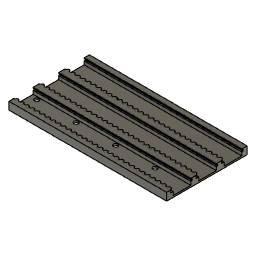
Plate Feeder for larger components v47 (Autodesk Fusion 360 design; units mm, degrees)
Autodesk Fusion 360 part; units mm, degrees
note: some values were not read from the file. Set by a fixed rule: which sketch regions a step uses.
sketch "Front view" plane through (0, 0, 0) normal (1, 0, 0) x (0, 1, 0)
  line L0 (0, 0) -> (16.4, 0)
  line L1 (16.4, 0) -> (16.4, 1.2)
  line L2 (16.4, 1.2) -> (0, 1.2)
  line L3 (0, 1.2) -> (0, 0)
  line L4 (0, 0) -> (-3, 0)
  line L5 (-3, 0) -> (-3, 5.8)
  line L6 (-3, 5.8) -> (0, 5.8)
  line L7 (0, 5.8) -> (0, 0)
  line L8 (16.4, 0) -> (19.4, 0)
  line L9 (19.4, 0) -> (19.4, 5.8)
  line L10 (19.4, 5.8) -> (16.4, 5.8)
  line L11 (16.4, 5.8) -> (16.4, 0)
  line L12 (0, 1.2) -> (16.4, 1.2)
  line L13 (16.4, 1.2) -> (16.4, 4.2) construction
  line L14 (16.4, 4.2) -> (0, 4.2) construction
  line L15 (0, 4.2) -> (0, 1.2) construction
  line L16 (16.4, 1.2) -> (15.4, 1.2)
  line L17 (15.4, 1.2) -> (15.4, 3.8)
  line L18 (15.4, 3.8) -> (16.4, 3.8)
  line L19 (16.4, 3.8) -> (16.4, 1.2)
  line L20 (0, 1.2) -> (2, 1.2)
  line L21 (2, 1.2) -> (2, 3.8)
  line L22 (2, 3.8) -> (0, 3.8)
  line L23 (0, 3.8) -> (0, 1.2)
  line L24 (35.8, 0) -> (35.8, 1.2)
  line L25 (35.8, 4.2) -> (19.4, 4.2) construction
  line L26 (35.8, 1.2) -> (34.8, 1.2)
  line L27 (35.8, 1.2) -> (35.8, 4.2) construction
  line L28 (34.8, 1.2) -> (34.8, 3.8)
  line L29 (21.4, 3.8) -> (19.4, 3.8)
  line L30 (38.8, 0) -> (38.8, 5.8)
  line L31 (19.4, 1.2) -> (21.4, 1.2)
  line L32 (21.4, 1.2) -> (21.4, 3.8)
  line L33 (35.8, 0) -> (38.8, 0)
  line L34 (34.8, 3.8) -> (35.8, 3.8)
  line L35 (35.8, 3.8) -> (35.8, 1.2)
  line L36 (38.8, 5.8) -> (35.8, 5.8)
  line L37 (35.8, 5.8) -> (35.8, 0)
  line L38 (35.8, 1.2) -> (19.4, 1.2)
  line L39 (19.4, 1.2) -> (35.8, 1.2)
  line L40 (19.4, 0) -> (35.8, 0)
  line L41 (55.2, 0) -> (55.2, 1.2)
  line L42 (55.2, 4.2) -> (38.8, 4.2) construction
  line L43 (55.2, 1.2) -> (54.2, 1.2)
  line L44 (55.2, 1.2) -> (55.2, 4.2) construction
  line L45 (54.2, 1.2) -> (54.2, 3.8)
  line L46 (40.8, 3.8) -> (38.8, 3.8)
  line L47 (58.2, 0) -> (58.2, 5.8)
  line L48 (38.8, 1.2) -> (40.8, 1.2)
  line L49 (40.8, 1.2) -> (40.8, 3.8)
  line L50 (55.2, 0) -> (58.2, 0)
  line L51 (54.2, 3.8) -> (55.2, 3.8)
  line L52 (55.2, 3.8) -> (55.2, 1.2)
  line L53 (58.2, 5.8) -> (55.2, 5.8)
  line L54 (55.2, 5.8) -> (55.2, 0)
  line L55 (55.2, 1.2) -> (38.8, 1.2)
  line L56 (38.8, 1.2) -> (55.2, 1.2)
  line L57 (38.8, 0) -> (55.2, 0)
  line L58 (0, 5.8) -> (2, 5.8)
  line L59 (2, 5.8) -> (2, 5.2)
  line L60 (2, 5.2) -> (0, 5.2)
  line L61 (0, 5.2) -> (0, 5.8)
  line L62 (16.4, 5.8) -> (15.4, 5.8)
  line L63 (15.4, 5.8) -> (15.4, 5.2)
  line L64 (15.4, 5.2) -> (16.4, 5.2)
  line L65 (16.4, 5.2) -> (16.4, 5.8)
  line L66 (34.8, 5.8) -> (34.8, 5.2)
  line L67 (35.8, 5.2) -> (35.8, 5.8)
  line L68 (35.8, 5.8) -> (34.8, 5.8)
  line L69 (34.8, 5.2) -> (35.8, 5.2)
  line L70 (21.4, 5.2) -> (19.4, 5.2)
  line L71 (19.4, 5.8) -> (21.4, 5.8)
  line L72 (21.4, 5.8) -> (21.4, 5.2)
  line L73 (54.2, 5.8) -> (54.2, 5.2)
  line L74 (55.2, 5.2) -> (55.2, 5.8)
  line L75 (55.2, 5.8) -> (54.2, 5.8)
  line L76 (54.2, 5.2) -> (55.2, 5.2)
  line L77 (40.8, 5.2) -> (38.8, 5.2)
  line L78 (38.8, 5.8) -> (40.8, 5.8)
  line L79 (40.8, 5.8) -> (40.8, 5.2)
  dimension "d8" = 16.4
  dimension "d9" = 1.2
  dimension "d11" = 3
  dimension "d12" = 5.8
  dimension "d14" = 3
  dimension "d15" = 5.8
  dimension "d17" = 16.4
  dimension "d18" = 3
  dimension "d20" = 1
  dimension "d21" = 2.6
  dimension "d22" = 2
  dimension "d23" = 2.6
  dimension "d33" = 38.8
  dimension "d34" = 0
  dimension "d65" = 2
  dimension "d66" = 0.6
  dimension "d67" = 1
  dimension "d68" = 0.6
  constraint horizontal L0
  constraint vertical L1
  constraint horizontal L2
  constraint vertical L3
  constraint coincident L0.start L3.end
  constraint horizontal L4
  constraint vertical L5
  constraint horizontal L6
  constraint vertical L7
  constraint horizontal L8
  constraint vertical L9
  constraint horizontal L10
  constraint vertical L11
  constraint horizontal L12
  constraint vertical L13
  constraint horizontal L14
  constraint vertical L15
  constraint horizontal L16
  constraint vertical L17
  constraint horizontal L18
  constraint vertical L19
  constraint horizontal L20
  constraint vertical L21
  constraint horizontal L22
  constraint vertical L23
  constraint horizontal L58
  constraint vertical L59
  constraint horizontal L60
  constraint vertical L61
  constraint horizontal L62
  constraint vertical L63
  constraint horizontal L64
  constraint vertical L65
  measures "d8" distance of L0.start L0.end
  measures "d9" distance of L0.start L2.end
  measures "d11" distance of L0.start L4.end
  measures "d12" distance of L0.start L6.end
  measures "d14" distance of L0.end L8.end
  measures "d15" distance of L0.end L10.end
  measures "d17" distance of L2.end L1.end
  measures "d18" distance of L2.end L14.end
  measures "d20" distance of L1.end L16.end
  measures "d21" distance of L1.end L18.end
  measures "d22" distance of L2.end L20.end
  measures "d23" distance of L2.end L22.end
  measures "d65" distance of L6.end L58.end
  measures "d66" distance of L6.end L60.end
  measures "d67" distance of L10.end L62.end
  measures "d68" distance of L10.end L64.end
extrude "Extrude4" add sketch "Front view" along normal blind 120
sketch "Mounting holes" plane through (0, 0, 0) normal (0, 0, 1) x (1, 0, 0)
  line L0 (0, 0) -> (5, 0) construction
  line L1 (5, 0) -> (5, 13.2) construction
  line L2 (5, 13.2) -> (0, 13.2) construction
  line L3 (0, 13.2) -> (0, 0) construction
  circle A0 centre (5, 13.2) radius 1.7
  line L4 (5, 13.2) -> (35, 13.2) construction
  line L5 (35, 13.2) -> (35, 43.2) construction
  line L6 (35, 43.2) -> (5, 43.2) construction
  line L7 (5, 43.2) -> (5, 13.2) construction
  circle A1 centre (35, 13.2) radius 1.7
  circle A2 centre (5, 43.2) radius 1.7
  circle A3 centre (35, 43.2) radius 1.7
  circle A4 centre (65, 43.2) radius 1.7
  circle A5 centre (65, 13.2) radius 1.7
  circle A6 centre (95, 43.2) radius 1.7
  circle A7 centre (95, 13.2) radius 1.7
  dimension "d37" = 5
  dimension "d38" = 13.2
  dimension "d40" = 3.4
  dimension "d41" = 30
  dimension "d42" = 30
  dimension "d45" = 30
  dimension "d46" = 30
  dimension "d83" = 60
  dimension "d84" = 0
  constraint horizontal L0
  constraint vertical L1
  constraint horizontal L2
  constraint vertical L3
  constraint coincident L0.start L3.end
  constraint coincident L1.end L2.start
  constraint horizontal L4
  constraint vertical L5
  constraint horizontal L6
  constraint vertical L7
  measures "d37" distance of L0.start L0.end
  measures "d38" distance of L0.start L2.end
  measures "d40" diameter of A0
  measures "d41" distance of L1.end L4.end
  measures "d42" distance of L1.end L6.end
extrude "Extrude5" cut sketch "Mounting holes" along normal blind 3
sketch "Tape holes" plane through (0, 0, 5.8) normal (0, 0, 1) x (-1, 0, 0)
  line L0 (0, -2) -> (0, 3)
  line L1 (0, 3) -> (-120, 3)
  line L2 (-120, 3) -> (-120, -2)
  line L3 (-120, -2) -> (0, -2)
  line L4 (0, 0) -> (0, -2) construction
  circle A0 centre (0, -2) radius 1.3
  circle A1 centre (-4, -2) radius 1.3
  circle A2 centre (-8, -2) radius 1.3
  circle A3 centre (-12, -2) radius 1.3
  circle A4 centre (-16, -2) radius 1.3
  circle A5 centre (-20, -2) radius 1.3
  circle A6 centre (-24, -2) radius 1.3
  circle A7 centre (-28, -2) radius 1.3
  circle A8 centre (-32, -2) radius 1.3
  circle A9 centre (-36, -2) radius 1.3
  circle A10 centre (-40, -2) radius 1.3
  circle A11 centre (0, -21.4) radius 1.3
  circle A12 centre (-4, -21.4) radius 1.3
  circle A13 centre (-8, -21.4) radius 1.3
  circle A14 centre (-12, -21.4) radius 1.3
  circle A15 centre (-16, -21.4) radius 1.3
  circle A16 centre (-20, -21.4) radius 1.3
  circle A17 centre (-24, -21.4) radius 1.3
  circle A18 centre (-28, -21.4) radius 1.3
  circle A19 centre (-32, -21.4) radius 1.3
  circle A20 centre (-36, -21.4) radius 1.3
  circle A21 centre (-40, -21.4) radius 1.3
  circle A22 centre (0, -40.8) radius 1.3
  circle A23 centre (-4, -40.8) radius 1.3
  circle A24 centre (-8, -40.8) radius 1.3
  circle A25 centre (-12, -40.8) radius 1.3
  circle A26 centre (-16, -40.8) radius 1.3
  circle A27 centre (-20, -40.8) radius 1.3
  circle A28 centre (-24, -40.8) radius 1.3
  circle A29 centre (-28, -40.8) radius 1.3
  circle A30 centre (-32, -40.8) radius 1.3
  circle A31 centre (-36, -40.8) radius 1.3
  circle A32 centre (-40, -40.8) radius 1.3
  circle A33 centre (-44, -2) radius 1.3
  circle A34 centre (-48, -2) radius 1.3
  circle A35 centre (-52, -2) radius 1.3
  circle A36 centre (-56, -2) radius 1.3
  circle A37 centre (-60, -2) radius 1.3
  circle A38 centre (-64, -2) radius 1.3
  circle A39 centre (-68, -2) radius 1.3
  circle A40 centre (-72, -2) radius 1.3
  circle A41 centre (-76, -2) radius 1.3
  circle A42 centre (-80, -2) radius 1.3
  circle A43 centre (-84, -2) radius 1.3
  circle A44 centre (-88, -2) radius 1.3
  circle A45 centre (-92, -2) radius 1.3
  circle A46 centre (-96, -2) radius 1.3
  circle A47 centre (-100, -2) radius 1.3
  circle A48 centre (-104, -2) radius 1.3
  circle A49 centre (-108, -2) radius 1.3
  circle A50 centre (-112, -2) radius 1.3
  circle A51 centre (-116, -2) radius 1.3
  circle A52 centre (-120, -2) radius 1.3
  circle A53 centre (-44, -21.4) radius 1.3
  circle A54 centre (-48, -21.4) radius 1.3
  circle A55 centre (-52, -21.4) radius 1.3
  circle A56 centre (-56, -21.4) radius 1.3
  circle A57 centre (-60, -21.4) radius 1.3
  circle A58 centre (-64, -21.4) radius 1.3
  circle A59 centre (-68, -21.4) radius 1.3
  circle A60 centre (-72, -21.4) radius 1.3
  circle A61 centre (-76, -21.4) radius 1.3
  circle A62 centre (-80, -21.4) radius 1.3
  circle A63 centre (-84, -21.4) radius 1.3
  circle A64 centre (-88, -21.4) radius 1.3
  circle A65 centre (-92, -21.4) radius 1.3
  circle A66 centre (-96, -21.4) radius 1.3
  circle A67 centre (-100, -21.4) radius 1.3
  circle A68 centre (-104, -21.4) radius 1.3
  circle A69 centre (-108, -21.4) radius 1.3
  circle A70 centre (-112, -21.4) radius 1.3
  circle A71 centre (-116, -21.4) radius 1.3
  circle A72 centre (-120, -21.4) radius 1.3
  circle A73 centre (-44, -40.8) radius 1.3
  circle A74 centre (-48, -40.8) radius 1.3
  circle A75 centre (-52, -40.8) radius 1.3
  circle A76 centre (-56, -40.8) radius 1.3
  circle A77 centre (-60, -40.8) radius 1.3
  circle A78 centre (-64, -40.8) radius 1.3
  circle A79 centre (-68, -40.8) radius 1.3
  circle A80 centre (-72, -40.8) radius 1.3
  circle A81 centre (-76, -40.8) radius 1.3
  circle A82 centre (-80, -40.8) radius 1.3
  circle A83 centre (-84, -40.8) radius 1.3
  circle A84 centre (-88, -40.8) radius 1.3
  circle A85 centre (-92, -40.8) radius 1.3
  circle A86 centre (-96, -40.8) radius 1.3
  circle A87 centre (-100, -40.8) radius 1.3
  circle A88 centre (-104, -40.8) radius 1.3
  circle A89 centre (-108, -40.8) radius 1.3
  circle A90 centre (-112, -40.8) radius 1.3
  circle A91 centre (-116, -40.8) radius 1.3
  circle A92 centre (-120, -40.8) radius 1.3
  dimension "d72" = 2
  dimension "d74" = 2.6
  dimension "d78" = -38.8
  constraint coincident L4.start origin
  constraint parallel L0 L4
  constraint coincident L0.start L3.end
  measures "d72" distance of L4.start L0.start
  measures "d74" diameter of A0
extrude "Extrude7" cut sketch "Tape holes" against normal blind 0.6 contours L0 L3 A0 | L0 L3 A0 | L3 A1 | L3 A1 | L2 L3 A52 | L2 L3 A52 | L3 A2 | L3 A2 | L3 A51 | L3 A51 | L3 A3 | L3 A3 | L3 A50 | L3 A50 | L3 A4 | L3 A4 | L3 A49 | L3 A49 | L3 A5 | L3 A5 | L3 A48 | L3 A48 | L3 A6 | L3 A6 | L3 A47 | L3 A47 | L3 A7 | L3 A7 | L3 A46 | L3 A46 | L3 A8 | L3 A8 | L3 A45 | L3 A45 | L3 A9 | L3 A9 | L3 A44 | L3 A44 | L3 A10 | L3 A10 | L3 A43 | L3 A43 | L3 A33 | L3 A33 | L3 A42 | L3 A42 | L3 A34 | L3 A34 | L3 A41 | L3 A41 | L3 A35 | L3 A35 | L3 A40 | L3 A40 | L3 A36 | L3 A36 | L3 A39 | L3 A39 | L3 A37 | L3 A37 | L3 A38 | L3 A38 | A11 | A12 | A13 | A14 | A15 | A16 | A17 | A18 | A19 | A20 | A21 | A22 | A23 | A24 | A25 | A26 | A27 | A28 | A29 | A30 | A31 | A32 | A53 | A54 | A55 | A56 | A57 | A58 | A59 | A60 | A61 | A62 | A63 | A64 | A65 | A66 | A67 | A68 | A69 | A70 | A71 | A72 | A73 | A74 | A75 | A76 | A77 | A78 | A79 | A80 | A81 | A82 | A83 | A84 | A85 | A86 | A87 | A88 | A89 | A90 | A91 | A92
equation "length = 120 mm" comment "Length of the feeder"
equation "number_positions = 3" comment "Number of feeder tapes next to each other"
equation "channel_width_clearance = 0.4 mm" comment "both sides included"
equation "channel_overhang_large = 2 mm" comment "for holding the tape in"
equation "wall_bottom = 1.2 mm" comment "height of the tape from the bottom where the tray is mounted"
equation "tape_width = 16 mm"
equation "d8 = tape_width + channel_width_clearance"
equation "d9 = wall_bottom"
equation "wall_width = 3 mm" comment "separator wall"
equation "d11 = wall_width"
equation "d12 = wall_height"
equation "wall_height = wall_bottom + tape_thickness + 1.6 mm" comment "separator height"
equation "d14 = wall_width"
equation "d15 = wall_height"
equation "tape_thickness = 3 mm"
equation "d17 = tape_width + channel_width_clearance"
equation "d18 = tape_thickness"
equation "channel_overhang_height = tape_thickness - 0.4 mm"
equation "d20 = channel_overhang_small"
equation "d21 = channel_overhang_height"
equation "d22 = channel_overhang_large"
equation "d23 = channel_overhang_height"
equation "mounting_holes_dist = 30 mm"
equation "d31 = number_positions"
equation "d33 = ( number_positions - 1 ) * ( wall_width + tape_width + channel_width_clearance )"
equation "mounting_hole_diam = 3.4 mm"
equation "d40 = mounting_hole_diam"
equation "d41 = mounting_holes_dist"
equation "d42 = mounting_holes_dist"
equation "d45 = mounting_holes_dist"
equation "d46 = mounting_holes_dist"
equation "d59 = length"
equation "d65 = channel_overhang_large"
equation "d66 = overhang_top_height"
equation "d67 = channel_overhang_small"
equation "d68 = overhang_top_height"
equation "channel_overhang_small = 1 mm"
equation "overhang_top_height = 0.6 mm"
equation "dist_between_holes_on_tape = 4 mm"
equation "d72 = channel_overhang_large"
equation "tape_hole_cutout_diam = 2.6 mm"
equation "d74 = tape_hole_cutout_diam"
equation "d75 = ( length / dist_between_holes_on_tape ) + 1"
equation "d76 = number_positions"
equation "d77 = -length"
equation "d78 = -( number_positions - 1 ) * ( tape_width + channel_width_clearance + wall_width )"
equation "d79 = -overhang_top_height"
equation "d83 = mounting_holes_dist * 2"
named bodies: "mm Feeder V"
